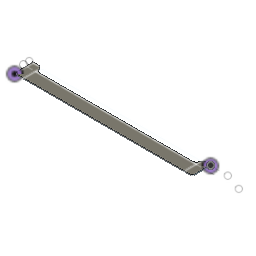
u1300L dash dimmer (Autodesk Fusion 360 design; units mm, degrees)
Autodesk Fusion 360 part; units mm, degrees
sketch "Sketch1" plane through (0, 0, 0) normal (0, 1, 0) x (1, 0, 0)
  line L0 (0, 0) -> (419.4969, 0)
  line L1 (419.4969, 0) -> (419.4969, 44.45)
  line L2 (419.4969, 44.45) -> (0, 44.45)
  line L3 (0, 44.45) -> (0, 0)
  line L4 (-8.9507, 43.45) -> (460, 43.45) construction
  line L5 (-8.9686, 29.45) -> (500, 29.45) construction
  line L6 (399.4969, 0) -> (399.4969, 44.45)
  line L7 (20, 44.45) -> (20, 0)
  line L8 (20, 29.45) -> (399.4969, 29.45)
  dimension "d1" = 419.4969
  dimension "d2" = 44.45
  dimension "d3" = 1
  dimension "d13" = 14
  dimension "d14" = 20
  dimension "d15" = 20
  constraint horizontal L0
  constraint vertical L1
  constraint horizontal L2
  constraint vertical L3
  constraint coincident L0.start L3.end
  constraint perpendicular L3 L4
  constraint perpendicular L1 L5
  constraint coincident L0 L6.start
  constraint coincident L2 L6.end
  constraint perpendicular L2 L6
  constraint coincident L2 L7.start
  constraint coincident L0 L7.end
  constraint perpendicular L0 L7
  constraint coincident L5 L8.start
  constraint coincident L7 L8.start
  constraint coincident L5 L8.end
  constraint coincident L6 L8.end
  measures "d1" distance of L0.start L0.end
  measures "d2" distance of L0.start L2.end
  measures "d3" distance of L2 L4
  measures "d13" distance of L4 L5
  measures "d14" distance of L1 L6
  measures "d15" distance of L3 L7
extrude "Extrude1" add sketch "Sketch1" along normal blind 2 contours L0 L2 L3 L7 | L0 L6 L7 L8 | L0 L1 L2 L6
sketch "Sketch2" plane through (419.4969, 0, 0) normal (1, 0, 0) x (0, 0, -1)
  line L0 (0, 0) -> (44.45, 0)
  line L1 (44.45, 0) -> (44.45, 2)
  line L2 (44.45, 2) -> (0, 2)
  line L3 (0, 2) -> (0, 0)
  line L4 (43.45, 0) -> (43.45, 2) construction
  circle A0 centre (43.45, 1) radius 1
  point P0 (43.45, 0)
  constraint coincident P0 L4.start
  constraint coincident L2 L4.end
  constraint perpendicular L2 L4
  constraint midpoint L4 A0.centre
  constraint coincident P0 A0
extrude "Extrude2" add sketch "Sketch2" along normal blind 2 contours A0
extrude "Extrude3" add sketch "Sketch2" against normal blind 2 from surface at -419.4969 contours A0
chamfer "Chamfer1" distance 5 angle 45 1 edges at (419.4969, 1, 0)
chamfer "Chamfer1" distance 5 angle 45 1 edges at (0, 1, 0)
fillet "Fillet1" radius 10 4 edges at (399.4969, 1, -44.45) (399.4969, 1, -29.45) (20, 1, -29.45) (20, 1, -44.45)
equation "d1 = 16 33/64\""
equation "d2 = 1 3/4\""
equation "d15 = d14"
